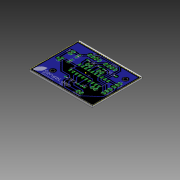
# Autodesk Inventor part: BOARD_IMAGE
Saved by Autodesk Inventor 2012 SP2 (Build 160219200, 219)
## iProperties
Created: 2013-02-23
Part Number: BOARD_IMAGE
Material: Default
Document SubType Name: Modeling
Designer: blacki
Density: 1 g/cm^3
Author: blacki
Autodesk Inventor part; units mm, degrees
ref_plane "YZ Plane" through (0, 0, 0) normal (1, 0, 0) x (0, 1, 0)
ref_plane "XZ Plane" through (0, 0, 0) normal (0, 1, 0) x (-1, 0, 0)
ref_plane "XY Plane" through (0, 0, 0) normal (0, 0, 1) x (1, 0, 0)
sketch "Sketch1" plane through (0, 0, 0) normal (0, 0, 1) x (1, 0, 0)
  line L0 (25, -20) -> (-25, -20)
  line L1 (-25, -20) -> (-25, 20)
  line L2 (-25, 20) -> (25, 20)
  line L3 (25, 20) -> (25, -20)
  line L4 (25, 0) -> (-25, 0) construction
  point P0 (0, 0)
  point P1 (0, 0)
  dimension "d0" = 50
  dimension "d1" = 40
  constraints: 10 end point, 3 midpoint, 2 parallel, 1 coincident, 1 horizontal, 1 perpendicular
  measures "d0" distance of L1.end L2.end
  measures "d1" distance of L0.end L1.end
extrude "Extrusion1" add sketch "Sketch1" along normal blind 1.6
sketch "Sketch2" plane through (0, 0, 1.6) normal (0, 0, 1) x (1, 0, 0)
  line L0 (-25, 18.8203) -> (25.4554, 18.8203) construction
  line L1 (25.4554, 18.8203) -> (25.4554, -19.9538) construction
  line L2 (25.4554, -19.9538) -> (-25, -19.9538) construction
  line L3 (-25, -19.9538) -> (-25, 18.8203) construction
  point P0 (0, 0)
  constraints: 2 other
sketch "Sketch3" plane through (0, 0, 1.6) normal (0, 0, 1) x (1, 0, 0)
  line L0 (-25, -20) -> (-25, 20) projected
  line L1 (25, -20) -> (-25, -20) projected
  point P0 (0, 0)
  point P1 (-15, -12)
  point P2 (20, 11)
  dimension "d5" = 8
  dimension "d6" = 10
  dimension "d7" = 45
  dimension "d8" = 31
  measures "d5" distance from line of L1 point (-15, -12)
  measures "d6" distance from line of L0 point (-15, -12)
  measures "d7" distance from line of L0 point (20, 11)
  measures "d8" distance from line of L1 point (20, 11)
hole "Hole1" at (20, 11, 1.6) at (-15, -12, 1.6) direction (0, 0, -1) diameter 3 end through all
body "Solid1"
